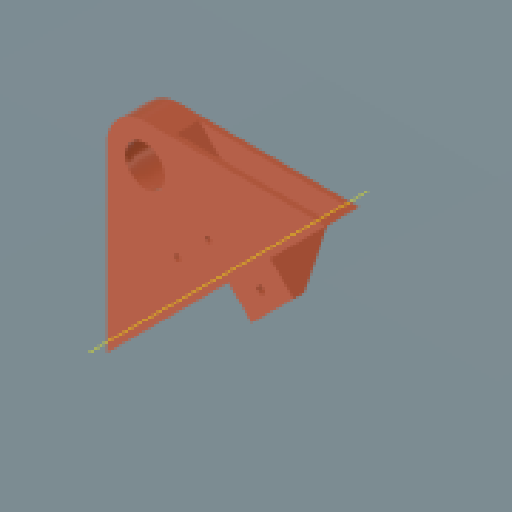
# Autodesk Inventor part: Rear Z Axis Bottom Bearing
Saved by Autodesk Inventor 2023.2 (Build 272271000, 271)
## iProperties
Created: 2023-02-18
Part Number: Rear Z Axis Bottom Bearing
Material: ABS Plastic
Document SubType Name: Modeling
Designer: remop
Density: 1.06 g/cm^3
Appearance: Smooth - Light Orange
Author: remop
Autodesk Inventor part; units mm, degrees
ref_plane "YZ Plane" through (0, 0, 0) normal (1, 0, 0) x (0, 1, 0)
ref_plane "XZ Plane" through (0, 0, 0) normal (0, 1, 0) x (-1, 0, 0)
ref_plane "XY Plane" through (0, 0, 0) normal (0, 0, 1) x (1, 0, 0)
sketch "Sketch1" plane through (0, 0, 0) normal (0, 0, 1) x (1, 0, 0)
  circle A0 centre (0, 0) radius 4 projected
  line L0 (-144.1925, -209.3609) -> (209.3609, 144.1925) projected
  circle A1 centre (0, 0) radius 11
  circle A2 centre (0, 0) radius 17.5
  line L1 (-17.5, 0) -> (-17.5, -82.6684)
  line L2 (0, 17.5) -> (82.6684, 17.5)
  point P0 (0, 0)
  dimension "d0" = 22
  dimension "d1" = 35
  constraints: 4 end point, 2 centre point, 2 coincident, 2 point on circle, 2 point on line, 2 tangent, 1 perpendicular, 1 vertical
  measures "d0" diameter of A1
  measures "d1" diameter of A2
extrude "Extrusion1" add sketch "Sketch1" against normal blind 15 contours L1 A2 L2 L0 | A2
sketch "Sketch2" plane through (0, 0, 0) normal (0, 0, 1) x (1, 0, 0)
  arc A0 (0, 17.5) -> (-17.5, 0) centre (0, 0) ccw projected
  line L0 (-17.5, 0) -> (-17.5, -82.6684) projected
  line L1 (-17.5, -82.6684) -> (82.6684, 17.5) projected
  line L2 (82.6684, 17.5) -> (0, 17.5) projected
  circle A1 centre (0, 0) radius 11 projected
  circle A2 centre (0, 0) radius 9
  dimension "d6" = 2
  constraints: 1 centre point, 1 coincident
  measures "d6" radial gap between concentric circles of A1 A2
extrude "Extrusion2" add sketch "Sketch2" against normal blind 3 contours A1
ref_plane "Work Plane1" through (-19.6213, -80.5471, 0) normal (0.7071068, -0.7071068, 0) x (-0.7071068, -0.7071068, 0)
sketch "Sketch3" plane through (-19.6213, -80.5471, 0) normal (0.7071068, -0.7071068, 0) x (-0.7071068, -0.7071068, 0)
  line L0 (-141.6595, 0) -> (-83.2041, 0) projected
  line L1 (-141.6595, 0) -> (-141.6595, 15) projected
  line L2 (-83.2041, 15) -> (-141.6595, 15) projected
  line L3 (-83.2041, 0) -> (-83.2041, 15) projected
  line L4 (-58.4554, 0) -> (0, 0) projected
  line L5 (-58.4554, 0) -> (-58.4554, 15) projected
  line L6 (0, 15) -> (-58.4554, 15) projected
  line L7 (0, 0) -> (0, 15) projected
  line L8 (-83.2041, 0) -> (-58.4554, 0) projected
  line L9 (-50.8297, 15) -> (-90.8297, 15) projected
  line L10 (-141.6595, 0) -> (-141.6595, 15) projected
  line L11 (-141.6595, 12.6) -> (-91.6595, 12.6)
  line L12 (-91.6595, 12.6) -> (-91.6595, 2.4)
  line L13 (-91.6595, 2.4) -> (-141.6595, 2.4)
  line L14 (-141.6595, 2.4) -> (-141.6595, 12.6)
  line L15 (0, 0) -> (0, 15) projected
  line L16 (0, 2.4) -> (-50, 2.4)
  line L17 (-50, 2.4) -> (-50, 12.6)
  line L18 (-50, 12.6) -> (0, 12.6)
  line L19 (0, 12.6) -> (0, 2.4)
  point P0 (-70.8297, 0)
  point P1 (0, 12.6)
  dimension "d8" = 2.4
  dimension "d9" = 2.4
  dimension "d10" = 2.4
  dimension "d11" = 50
  constraints: 16 end point, 4 parallel, 3 point on line, 2 horizontal, 2 perpendicular, 1 collinear
  measures "d8" distance between parallel lines of L2 L11
  measures "d9" distance between parallel lines of L0 L13
  measures "d10" distance between parallel lines of L4 L16
  measures "d11" distance of L17.end L18.end
extrude "Extrusion3" cut sketch "Sketch3" against normal through all contours L1 L11 L12 L13 | L16 L17 L18 L7
sketch "Sketch4" plane through (-19.6213, -80.5471, 0) normal (-0.7071068, 0.7071068, 0) x (0, 0, 1)
  line L0 (-12.6, 138.6595) -> (-2.4, 138.6595) projected
  line L1 (-12.6, 91.6595) -> (-12.6, 138.6595) projected
  line L2 (-2.4, 91.6595) -> (-12.6, 91.6595) projected
  line L3 (-2.4, 138.6595) -> (-2.4, 91.6595) projected
  line L4 (-2.4, 3) -> (-12.6, 3) projected
  line L5 (-2.4, 50) -> (-2.4, 3) projected
  line L6 (-12.6, 50) -> (-2.4, 50) projected
  line L7 (-12.6, 3) -> (-12.6, 50) projected
  line L8 (-12.6, 50) -> (-2.4, 50) projected
  line L9 (-2.4, 91.6595) -> (-12.6, 91.6595) projected
  point P0 (0, 70.8297)
  point P1 (-7.5, 106.6595)
  point P2 (-7.5, 126.6595)
  point P3 (-7.5, 35)
  point P4 (-7.5, 15)
  point P5 (-7.5, 50)
  point P6 (-7.5, 91.6595)
  dimension "d14" = 15
  dimension "d15" = 15
  dimension "d16" = 20
  dimension "d17" = 20
  constraints: 4 vertical alignment, 2 midpoint
  measures "d14" distance from line of L2 point (-7.5, 106.659)
  measures "d15" distance from line of point (-7.5, 35) L6
  measures "d16" distance of point (-7.5, 126.659) point (-7.5, 106.659)
  measures "d17" distance of point (-7.5, 35) point (-7.5, 15)
hole "Hole1" at (55.7983, -5.1274, -7.5) at (69.9405, 9.0147, -7.5) at (5.1274, -55.7983, -7.5) at (-9.0147, -69.9405, -7.5) direction (0.7071068, -0.7071068, 0) diameter 3.6 end through all clearance for "Hex Head Cap Screw DIN EN 24017" size "M3" standard "DIN"
sketch "Sketch5" plane through (0, 0, 0) normal (0, 0, 1) x (1, 0, 0)
  circle A0 centre (0, 0) radius 9 projected
  arc A1 (0, 17.5) -> (-17.5, 0) centre (0, 0) ccw projected
  line L0 (-17.5, 0) -> (-17.5, -82.6684) projected
  line L1 (-17.5, -82.6684) -> (82.6684, 17.5) projected
  line L2 (82.6684, 17.5) -> (0, 17.5) projected
  line L3 (29, -14.8579) -> (14.8579, -29) construction
  dimension "d25" = 29
  dimension "d26" = 29
  dimension "d27" = 20
  constraints: 2 end point, 1 parallel
  measures "d25" horizontal distance of L3.start point (0, 0)
  measures "d26" vertical distance of point (0, 0) L3.end
  measures "d27" distance of L3.end L3.start
hole "Hole2" at (29, -14.8579, 0) at (14.8579, -29, 0) direction (0, 0, -1) diameter 2.9 end through all
sketch "Sketch6" plane through (0, 0, -15) normal (0, 0, -1) x (-1, 0, 0)
  circle A0 centre (-29, -14.8579) radius 1.45 projected
  circle A1 centre (-14.8579, -29) radius 1.45 projected
  arc A2 (17.5, 0) -> (0, 17.5) centre (0, 0) ccw projected
  line L0 (0, 17.5) -> (-82.6684, 17.5) projected
  line L1 (-82.6684, 17.5) -> (17.5, -82.6684) projected
  line L2 (17.5, -82.6684) -> (17.5, 0) projected
  circle A3 centre (0, 0) radius 11 projected
  circle A4 centre (-14.8579, -29) radius 1.45 projected
  circle A5 centre (-14.8579, -29) radius 3.5
  circle A6 centre (-29, -14.8579) radius 1.45 projected
  circle A7 centre (-29, -14.8579) radius 3.5
  line L3 (-12.383, -31.4749) -> (-23.0382, -42.1301)
  line L4 (-17.3327, -26.5251) -> (-27.988, -37.1804)
  line L5 (-82.6684, 17.5) -> (17.5, -82.6684) projected
  line L6 (-31.4749, -12.383) -> (-42.1301, -23.0382)
  line L7 (-26.5251, -17.3327) -> (-37.1804, -27.988)
  point P0 (0, 0)
  dimension "d35" = 7
  constraints: 8 end point, 4 perpendicular, 4 point on circle, 4 point on line, 4 tangent, 2 centre point, 2 coincident, 1 equal radius
  measures "d35" diameter of A5
extrude "Extrusion4" add sketch "Sketch6" along normal blind 26 contours L1 L4 A5 L3 | L6 A7 L7 L1 | A5 | A7
sketch "Sketch7" plane through (0, 0, -15) normal (0, 0, -1) x (-1, 0, 0)
  line L0 (-26.5251, -17.3327) -> (-37.1804, -27.988) projected
  line L1 (-37.1804, -27.988) -> (-27.988, -37.1804) projected
  line L2 (-27.988, -37.1804) -> (-17.3327, -26.5251) projected
  arc A0 (-12.383, -31.4749) -> (-17.3327, -26.5251) centre (-14.8579, -29) ccw projected
  line L3 (-12.383, -31.4749) -> (-23.0382, -42.1301) projected
  line L4 (-23.0382, -42.1301) -> (17.5, -82.6684) projected
  line L5 (17.5, -82.6684) -> (17.5, 0) projected
  arc A1 (17.5, 0) -> (0, 17.5) centre (0, 0) ccw projected
  line L6 (0, 17.5) -> (-82.6684, 17.5) projected
  line L7 (-82.6684, 17.5) -> (-42.1301, -23.0382) projected
  line L8 (-42.1301, -23.0382) -> (-31.4749, -12.383) projected
  arc A2 (-26.5251, -17.3327) -> (-31.4749, -12.383) centre (-29, -14.8579) ccw projected
  circle A3 centre (0, 0) radius 11 projected
  line L9 (-12.383, -26.5251) -> (-26.5251, -12.383)
  arc A4 (-26.5251, -17.3327) -> (-31.4749, -12.383) centre (-29, -14.8579) ccw projected
  point P0 (0, 0)
  constraints: 3 point on circle, 2 end point
extrude "Extrusion5" add sketch "Sketch7" along normal blind 23 contours A2 L9 A0 L2 L1 L0
sketch "Sketch8" plane through (-17.5, -82.6684, 0) normal (0.7071068, -0.7071068, 0) x (-0.7071068, -0.7071068, 0)
  circle A0 centre (-35, 7.5) radius 1.8 projected
  circle A1 centre (-106.6595, 7.5) radius 1.8 projected
  circle A2 centre (-126.6595, 7.5) radius 1.8 projected
  circle A3 centre (-15, 7.5) radius 1.8 projected
  line L0 (0, 0) -> (-141.6595, 0) projected
  line L1 (0, 0) -> (0, 15) projected
  line L2 (-57.3297, 15) -> (0, 15) projected
  line L3 (-57.3297, 15) -> (-57.3297, 41) projected
  line L4 (-64.3297, 41) -> (-57.3297, 41) projected
  line L5 (-64.3297, 38) -> (-64.3297, 41) projected
  line L6 (-77.3297, 38) -> (-64.3297, 38) projected
  line L7 (-77.3297, 38) -> (-77.3297, 41) projected
  line L8 (-84.3297, 41) -> (-77.3297, 41) projected
  line L9 (-84.3297, 15) -> (-84.3297, 41) projected
  line L10 (-141.6595, 15) -> (-84.3297, 15) projected
  line L11 (-141.6595, 0) -> (-141.6595, 15) projected
  line L12 (-84.3297, 15) -> (-57.3297, 15)
  line L13 (-83.2041, 15) -> (-141.6595, 15) projected
  line L14 (-84.3297, 15) -> (-84.3297, 41) projected
  line L15 (-84.3297, 20) -> (-57.3297, 20)
  point P0 (-70.8297, 0)
  dimension "d40" = 5
  constraints: 4 end point, 2 point on line, 1 collinear, 1 perpendicular
  measures "d40" distance between parallel lines of L12 L15
extrude "Extrusion6" add sketch "Sketch8" along normal blind 15 contours L12 L9 L15 L3
sketch "Sketch9" plane through (31.4749, -12.383, -41) normal (0.7071068, 0.7071068, 0) x (-0.7071068, 0.7071068, 0)
  line L0 (-15.0688, 26) -> (0, 26) projected
  line L1 (-15.0688, 26) -> (-30.0688, 26) projected
  line L2 (-30.0688, 21) -> (-30.0688, 26) projected
  line L3 (-15.0688, 21) -> (-30.0688, 21) projected
  line L4 (-15.0688, 21) -> (-15.0688, 0) projected
  line L5 (0, 0) -> (-15.0688, 0) projected
  line L6 (0, 26) -> (0, 0) projected
  line L7 (-15.0688, 0) -> (-30.0688, 21)
  point P0 (31.0122, 41)
  constraints: 2 end point
extrude "Extrusion7" add sketch "Sketch9" against normal blind 5 contours L3 L4 L7
sketch "Sketch10" plane through (12.383, -31.4749, -15) normal (-0.7071068, -0.7071068, 0) x (-0.7071068, 0.7071068, 0)
  line L0 (-15.0688, 26) -> (-30.0688, 5) projected
  line L1 (-15.0688, 5) -> (-30.0688, 5) projected
  line L2 (-15.0688, 26) -> (-15.0688, 5) projected
  point P0 (31.0122, -15)
extrude "Extrusion8" add sketch "Sketch10" against normal blind 5
sketch "Sketch11" plane through (49.2012, -37.1804, -20) normal (0, 0, -1) x (-0.7071068, -0.7071068, 0)
  line L0 (17, 0) -> (17, 15) projected
  line L1 (0, 15) -> (17, 15) projected
  line L2 (0, 15) -> (0, 0) projected
  line L3 (17, 0) -> (0, 0) projected
  line L4 (2, 15) -> (15, 15) projected
  point P0 (8.5, 61.081)
  point P1 (8.5, 7.5)
  point P2 (0, 7.5)
  point P3 (8.5, 15)
  constraints: 2 midpoint, 1 horizontal alignment, 1 vertical alignment
hole "Hole3" at (37.8875, -37.8875, -20) direction (0, 0, 1) diameter 3.5 end through all
equation "\"d9\" = d8"
equation "\"d10\" = d8"
equation "\"d15\" = d14"
equation "\"d17\" = d16"
equation "\"d26\" = d25"
body "Solid1"
